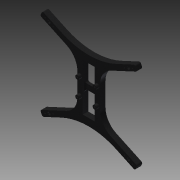
# Autodesk Inventor part: micro_h-quad-naze
Saved by Autodesk Inventor 2014 (Build 180170000, 170)
## iProperties
Created: 2013-01-19
Part Number: micro_h-quad-naze
Material: Plastique ABS
Document SubType Name: Modeling
Designer: Army
Density: 1.06 g/cm^3
Mass: 59.4442 g
Surface Area: 227.74 cm^2
Volume: 56.0794 cm^3
Appearance: Moulé noir
Author: Army
Autodesk Inventor part; units mm, degrees
ref_plane "YZ Plane" through (0, 0, 0) normal (1, 0, 0) x (0, 1, 0)
ref_plane "XZ Plane" through (0, 0, 0) normal (0, 1, 0) x (-1, 0, 0)
ref_plane "XY Plane" through (0, 0, 0) normal (0, 0, 1) x (1, 0, 0)
sketch "Sketch1" plane through (0, 0, 0) normal (0, 1, 0) x (-1, 0, 0)
  line L0 (-69.85, 69.85) -> (69.85, 69.85) construction
  line L1 (69.85, 69.85) -> (69.85, -69.85) construction
  line L2 (69.85, -69.85) -> (-69.85, -69.85) construction
  line L3 (-69.85, -69.85) -> (-69.85, 69.85) construction
  line L4 (-15.25, 69.85) -> (-15.25, -69.85) construction
  line L5 (15.25, 69.85) -> (15.25, -69.85) construction
  line L6 (-69.85, 0) -> (69.85, 0) construction
  line L7 (0, 69.85) -> (0, -69.85) construction
  line L8 (-10.4875, 41.5925) -> (-10.4875, -41.5925)
  line L9 (10.4875, 41.5925) -> (10.4875, -41.5925)
  circle A0 centre (-69.85, 69.85) radius 2.5
  circle A1 centre (69.85, 69.85) radius 2.5
  circle A2 centre (69.85, -69.85) radius 2.5
  circle A3 centre (-69.85, -69.85) radius 2.5
  line L10 (-15.25, 15.25) -> (15.25, 15.25) construction
  line L11 (-15.25, -15.25) -> (15.25, -15.25) construction
  circle A4 centre (-15.25, 15.25) radius 1.25
  circle A5 centre (15.25, 15.25) radius 1.25
  circle A6 centre (15.25, -15.25) radius 1.25
  circle A7 centre (-15.25, -15.25) radius 1.25
  line L12 (-69.85, 69.85) -> (-28.5605, 50.5964) construction
  line L13 (69.85, 69.85) -> (28.5605, 50.5964) construction
  line L14 (-69.85, -69.85) -> (-28.5605, -50.5964) construction
  line L15 (69.85, -69.85) -> (28.5605, -50.5964) construction
  line L16 (-85.4573, 71.873) -> (-20.0125, 41.3556)
  line L17 (-81.4319, 80.5056) -> (-18.409, 51.1175)
  line L18 (-85.4573, 71.873) -> (-81.4319, 80.5056)
  line L19 (85.4573, 71.873) -> (20.0125, 41.3556)
  line L20 (81.4319, 80.5056) -> (18.409, 51.1175)
  line L21 (85.4573, 71.873) -> (81.4319, 80.5056)
  line L22 (-85.4573, -71.873) -> (-20.0125, -41.3556)
  line L23 (-81.4319, -80.5056) -> (-18.409, -51.1175)
  line L24 (-85.4573, -71.873) -> (-81.4319, -80.5056)
  line L25 (85.4573, -71.873) -> (20.0125, -41.3556)
  line L26 (81.4319, -80.5056) -> (18.409, -51.1175)
  line L27 (85.4573, -71.873) -> (81.4319, -80.5056)
  line L28 (-18.409, 51.1175) -> (18.409, 51.1175)
  line L29 (-18.409, -51.1175) -> (18.409, -51.1175)
  circle A8 centre (-76.9328, 73.1528) radius 1
  circle A9 centre (-62.7672, 66.5472) radius 1
  circle A10 centre (76.9328, 73.1528) radius 1
  circle A11 centre (62.7672, 66.5472) radius 1
  circle A12 centre (-76.9328, -73.1528) radius 1
  circle A13 centre (-62.7672, -66.5472) radius 1
  circle A14 centre (76.9328, -73.1528) radius 1
  circle A15 centre (62.7672, -66.5472) radius 1
  line L30 (-20.0125, 41.3556) -> (-20.0125, -41.3556)
  line L31 (20.0125, 41.3556) -> (20.0125, -41.3556)
  line L32 (-10.4875, -41.5925) -> (10.4875, -41.5925)
  line L33 (-10.4875, 41.5925) -> (10.4875, 41.5925)
  point P0 (0, 0)
  dimension "d0" = 139.7
  dimension "d2" = 139.7
  dimension "d3" = 69.85
  dimension "d4" = 69.85
  dimension "d5" = 30.5
  dimension "d6" = 15.25
  dimension "d9" = 4.7625
  dimension "d11" = 5
  dimension "d12" = 5
  dimension "d13" = 5
  dimension "d14" = 5
  dimension "d15" = 30.5
  dimension "d16" = 15.25
  dimension "d17" = 2.5
  dimension "d18" = 2.5
  dimension "d19" = 2.5
  dimension "d20" = 2.5
  dimension "d21" = 25
  dimension "d22" = 9.525
  dimension "d23" = 4.7625
  dimension "d24" = 15
  dimension "d25" = 15.63
  dimension "d26" = 7.815
  dimension "d27" = 2
  dimension "d28" = 2
  dimension "d52" = 83.185
  dimension "d55" = 9.525
  dimension "d56" = 9.525
  dimension "d57" = 41.5925
  dimension "d58" = 9.525
  constraints: 68 end point, 24 symmetric about line, 16 centre point, 10 point on line, 9 parallel, 9 perpendicular, 8 coincident, 4 midpoint, 1 horizontal, 6 other
  measures "d0" distance of L1.end L2.end
  measures "d2" distance of L2.end L0.start
  measures "d3" distance from line of point (0, 0) L3
  measures "d4" distance from line of point (0, 0) L0
  measures "d5" distance between parallel lines of L4 L5
  measures "d6" distance from line of point (0, 0) L4
  measures "d9" distance between parallel lines of L5 L9
  measures "d11" diameter of A0
  measures "d12" diameter of A1
  measures "d13" diameter of A2
  measures "d14" diameter of A3
  measures "d15" distance between parallel lines of L11 L10
  measures "d16" distance from line of point (0, 0) L10
  measures "d17" diameter of A4
  measures "d18" diameter of A5
  measures "d19" diameter of A6
  measures "d20" diameter of A7
  measures "d21" angle of L0 L12
  measures "d22" distance between parallel lines of L17 L16
  measures "d23" distance between parallel lines of L12 L16
  measures "d24" distance from line of L0.start L18
  measures "d25" distance of A9.centre A8.centre
  measures "d26" distance of L0.start A9.centre
  measures "d27" diameter of A9
  measures "d28" diameter of A8
  measures "d52" distance between parallel lines of L32 L33
  measures "d55" distance between parallel lines of L31 L9
  measures "d56" distance between parallel lines of L8 L30
  measures "d57" distance between parallel lines of L6 L33
  measures "d58" distance between parallel lines of L29 L32
extrude "Extrusion1" add sketch "Sketch1" along normal blind 9.525
sketch "Sketch2" plane through (0, 9.525, 0) normal (0, 1, 0) x (1, 0, 0)
  circle A0 centre (15.25, 15.25) radius 1.25 projected
  circle A1 centre (-15.25, 15.25) radius 1.25 projected
  circle A2 centre (-15.25, -15.25) radius 1.25 projected
  circle A3 centre (15.25, -15.25) radius 1.25 projected
  circle A4 centre (-15.25, 15.25) radius 3.5
  circle A5 centre (15.25, 15.25) radius 3.5
  circle A6 centre (15.25, -15.25) radius 3.5
  circle A7 centre (-15.25, -15.25) radius 3.5
  point P0 (0, 0)
  dimension "d31" = 7
  dimension "d34" = 7
  dimension "d35" = 7
  dimension "d36" = 7
  constraints: 4 centre point, 4 coincident
  measures "d31" diameter of A7
  measures "d34" diameter of A6
  measures "d35" diameter of A4
  measures "d36" diameter of A5
extrude "Extrusion2" add sketch "Sketch2" along normal blind 5
sketch "Sketch3" plane through (0, 0, 0) normal (0, -1, 0) x (1, 0, 0)
  circle A0 centre (15.25, -15.25) radius 1.25 projected
  circle A1 centre (-15.25, -15.25) radius 1.25 projected
  circle A2 centre (-15.25, 15.25) radius 1.25 projected
  circle A3 centre (15.25, 15.25) radius 1.25 projected
  point P0 (0, 0)
extrude "Extrusion3" add sketch "Sketch3" against normal blind 9.525
sketch "Sketch4" plane through (0, 0, 0) normal (0, -1, 0) x (1, 0, 0)
  circle A0 centre (69.85, -69.85) radius 2.5 projected
  circle A1 centre (-69.85, -69.85) radius 2.5 projected
  circle A2 centre (-69.85, 69.85) radius 2.5 projected
  circle A3 centre (69.85, 69.85) radius 2.5 projected
  circle A4 centre (-76.9328, -73.1528) radius 1 projected
  circle A5 centre (-62.7672, -66.5472) radius 1 projected
  circle A6 centre (62.7672, -66.5472) radius 1 projected
  circle A7 centre (76.9328, -73.1528) radius 1 projected
  circle A8 centre (-62.7672, 66.5472) radius 1 projected
  circle A9 centre (-76.9328, 73.1528) radius 1 projected
  circle A10 centre (62.7672, 66.5472) radius 1 projected
  circle A11 centre (76.9328, 73.1528) radius 1 projected
  point P0 (0, 0)
extrude "Extrusion4" add sketch "Sketch4" against normal blind 4.7625
sketch "Sketch5" plane through (0, 0, 0) normal (0, -1, 0) x (1, 0, 0)
  line L0 (10.4875, 41.5925) -> (10.4875, -41.5925) projected
  line L1 (-10.4875, -41.5925) -> (-10.4875, 41.5925) projected
  line L2 (-10.4875, -4.7625) -> (10.4875, -4.7625)
  line L3 (10.4875, -4.7625) -> (10.4875, 4.7625)
  line L4 (10.4875, 4.7625) -> (-10.4875, 4.7625)
  line L5 (-10.4875, 4.7625) -> (-10.4875, -4.7625)
  point P0 (0, 0)
  dimension "d43" = 9.525
  dimension "d45" = 4.7625
  constraints: 8 end point, 2 parallel, 2 point on line, 1 horizontal, 1 perpendicular
  measures "d43" distance between parallel lines of L2 L4
  measures "d45" distance from line of L4 point (0, 0)
extrude "Extrusion5" add sketch "Sketch5" against normal blind 4.7625
fillet "Fillet1" radius 114.3 4 edges at (18.409, 4.7625, -51.1175) (-18.409, 4.7625, -51.1175) (-18.409, 4.7625, 51.1175) (18.409, 4.7625, 51.1175)
fillet "Fillet2" radius 3.175 6 edges at (10.4875, 2.3813, 4.7625) (10.4875, 4.7625, 0) (10.4875, 2.3813, -4.7625) (-10.4875, 4.7625, 0) (-10.4875, 2.3813, -4.7625) (-10.4875, 2.3813, 4.7625)
fillet "Fillet3" radius 33.02 4 edges at (-20.0125, 4.7625, 41.3556) (-20.0125, 4.7625, -41.3556) (20.0125, 4.7625, 41.3556) (20.0125, 4.7625, -41.3556)
fillet "Fillet5" radius 2.54 8 edges at (81.4319, 4.7625, 80.5056) (85.4573, 4.7625, 71.873) (85.4573, 4.7625, -71.873) (81.4319, 4.7625, -80.5056) (-85.4573, 4.7625, 71.873) (-81.4319, 4.7625, 80.5056) (-81.4319, 4.7625, -80.5056) (-85.4573, 4.7625, -71.873)
move or copy body "Déplacer des corps1" bodies to move or copy 1 copy no rotation origin (0, 0, 0) rotation axis (1, 0, 0) rotation angle 90
body "Solid1"
